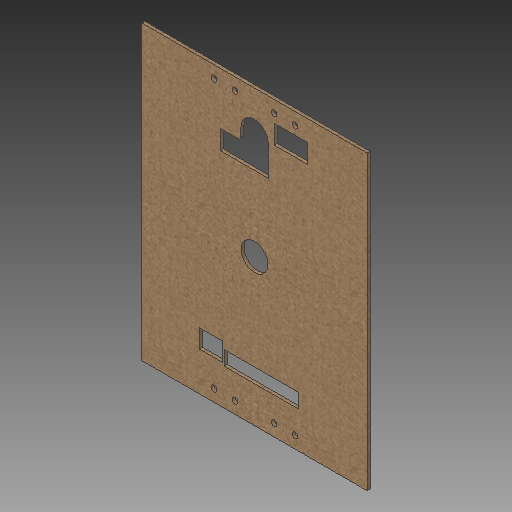
# Autodesk Inventor part: 基板保護2018.8.7
Saved by Autodesk Inventor 2018 (Build 220112000, 112)
## iProperties
Created: 2018-08-07
Part Number: 基板保護2018.8.7
Material: MDF 中密度繊維ボード
Document SubType Name: Modeling
Designer: shun2
Density: 0.8 g/cm^3
Appearance: ダンボール - 段ボール紙
Author: shun2
Autodesk Inventor part; units mm, degrees
(part 1 of 2)
ref_plane "YZ Plane" through (0, 0, 0) normal (1, 0, 0) x (0, 1, 0)
ref_plane "XZ Plane" through (0, 0, 0) normal (0, 1, 0) x (-1, 0, 0)
ref_plane "XY Plane" through (0, 0, 0) normal (0, 0, 1) x (1, 0, 0)
sketch "スケッチ1" plane through (0, 0, 0) normal (0, 0, 1) x (1, 0, 0)
  line L0 (-10, 0) -> (140, 0)
  arc A0 (140, -0.0003) -> (140, 0.0003) centre (140, 0) ccw
  arc A1 (-10, 0.0003) -> (-10, -0.0003) centre (-10, 0) ccw
  line L1 (140, 0) -> (140, 194.7239)
  arc A2 (140.0002, 194.7239) -> (139.9998, 194.7239) centre (140, 194.7239) ccw
  arc A3 (139.9998, 0) -> (140.0002, 0) centre (140, 0) ccw
  line L2 (140, 194.7239) -> (-10, 194.7239)
  arc A4 (-10, 194.7242) -> (-10, 194.7237) centre (-10, 194.72395) ccw
  arc A5 (140, 194.7237) -> (140, 194.7242) centre (140, 194.72395) ccw
  line L3 (-10, 194.7239) -> (-10, 0)
  arc A6 (-10.0002, 0) -> (-9.9998, 0) centre (-10, 0) ccw
  arc A7 (-9.9998, 194.7239) -> (-10.0002, 194.7239) centre (-10, 194.7239) ccw
  arc A8 (65, 88.362) -> (65, 106.362) centre (65, 97.362) ccw
  arc A9 (65, 106.362) -> (65, 88.362) centre (65, 97.362) ccw
  line L4 (89.7664, 26.5952) -> (89.6098, 26.5952)
  arc A10 (89.6098, 26.6143) -> (89.6098, 26.5762) centre (89.6098, 26.59525) ccw
  arc A11 (89.7664, 26.5762) -> (89.7664, 26.6143) centre (89.7664, 26.59525) ccw
  line L5 (89.6098, 26.5952) -> (89.6098, 26.0731)
  arc A12 (89.5907, 26.0731) -> (89.6288, 26.0731) centre (89.60975, 26.0731) ccw
  arc A13 (89.6288, 26.5952) -> (89.5907, 26.5952) centre (89.60975, 26.5952) ccw
  line L6 (89.6098, 26.0731) -> (89.9231, 26.0731)
  arc A14 (89.9231, 26.0541) -> (89.9231, 26.0922) centre (89.9231, 26.07315) ccw
  arc A15 (89.6098, 26.0922) -> (89.6098, 26.0541) centre (89.6098, 26.07315) ccw
  arc A16 (89.9231, 26.0731) -> (90.1319, 26.2819) centre (89.923095, 26.281905) ccw
  arc A17 (89.9231, 26.0922) -> (89.9231, 26.0541) centre (89.9231, 26.07315) ccw
  arc A18 (90.1509, 26.2819) -> (90.1129, 26.2819) centre (90.1319, 26.2819) ccw
  line L7 (90.1319, 26.2819) -> (90.1319, 26.8041)
  arc A19 (90.1509, 26.8041) -> (90.1129, 26.8041) centre (90.1319, 26.8041) ccw
  arc A20 (90.1129, 26.2819) -> (90.1509, 26.2819) centre (90.1319, 26.2819) ccw
  arc A21 (90.1319, 26.8041) -> (89.9231, 27.0129) centre (89.923095, 26.804095) ccw
  arc A22 (90.1129, 26.8041) -> (90.1509, 26.8041) centre (90.1319, 26.8041) ccw
  arc A23 (89.9231, 27.0319) -> (89.9231, 26.9938) centre (89.9231, 27.01285) ccw
  line L8 (89.9231, 27.0129) -> (89.6098, 27.0129)
  arc A24 (89.6098, 27.032) -> (89.6098, 26.9939) centre (89.6098, 27.01295) ccw
  arc A25 (89.9231, 26.9939) -> (89.9231, 27.032) centre (89.9231, 27.01295) ccw
  arc A26 (84.5298, 26.2819) -> (84.7386, 26.0731) centre (84.738605, 26.281905) ccw
  arc A27 (84.5488, 26.2819) -> (84.5107, 26.2819) centre (84.52975, 26.2819) ccw
  arc A28 (84.7386, 26.0541) -> (84.7386, 26.0922) centre (84.7386, 26.07315) ccw
  arc A29 (84.7386, 26.0731) -> (85.0519, 26.2036) centre (84.73865, 26.51431) ccw
  arc A30 (84.7386, 26.0921) -> (84.7386, 26.0541) centre (84.7386, 26.0731) ccw
  arc A31 (85.0654, 26.1902) -> (85.0384, 26.217) centre (85.0519, 26.2036) ccw
  arc A32 (85.0258, 26.8041) -> (84.817, 27.0129) centre (84.816995, 26.804095) ccw
  arc A33 (85.0067, 26.8041) -> (85.0448, 26.8041) centre (85.02575, 26.8041) ccw
  arc A34 (84.817, 27.032) -> (84.817, 26.9939) centre (84.817, 27.01295) ccw
  arc A35 (84.817, 27.0129) -> (84.582, 26.9346) centre (84.816933, 26.621301) ccw
  arc A36 (84.817, 26.9939) -> (84.8169, 27.032) centre (84.81695, 27.01295) ccw
  arc A37 (84.5706, 26.9498) -> (84.5934, 26.9193) centre (84.582, 26.93455) ccw
  arc A38 (84.9214, 26.6213) -> (85.0258, 26.8041) centre (84.813675, 26.804036) ccw
  arc A39 (84.9117, 26.6377) -> (84.931, 26.6049) centre (84.92135, 26.6213) ccw
  arc A40 (85.0448, 26.8041) -> (85.0067, 26.8041) centre (85.02575, 26.8041) ccw
  arc A41 (84.6342, 26.4647) -> (84.5298, 26.2819) centre (84.741925, 26.281964) ccw
  arc A42 (84.6439, 26.4483) -> (84.6245, 26.4811) centre (84.6342, 26.4647) ccw
  arc A43 (84.5107, 26.2819) -> (84.5488, 26.2819) centre (84.52975, 26.2819) ccw
  line L9 (84.6342, 26.4647) -> (84.9214, 26.6213)
  arc A44 (84.9305, 26.6046) -> (84.9123, 26.638) centre (84.9214, 26.6213) ccw
  arc A45 (84.6251, 26.4814) -> (84.6433, 26.448) centre (84.6342, 26.4647) ccw
  line L10 (84.0898, 27.0129) -> (84.0898, 26.0731)
  arc A46 (84.0708, 26.0731) -> (84.1089, 26.0731) centre (84.08985, 26.0731) ccw
  arc A47 (84.1089, 27.0129) -> (84.0708, 27.0129) centre (84.08985, 27.0129) ccw
  line L11 (84.1942, 26.0731) -> (83.9854, 26.0731)
  arc A48 (83.9854, 26.0922) -> (83.9854, 26.0541) centre (83.9854, 26.07315) ccw
  arc A49 (84.1942, 26.0541) -> (84.1942, 26.0922) centre (84.1942, 26.07315) ccw
  line L12 (84.1942, 27.0129) -> (83.9854, 27.0129)
  arc A50 (83.9854, 27.032) -> (83.9854, 26.9939) centre (83.9854, 27.01295) ccw
  arc A51 (84.1942, 26.9939) -> (84.1942, 27.032) centre (84.1942, 27.01295) ccw
  line L13 (83.2234, 26.5952) -> (83.0668, 26.5952)
  arc A52 (83.0668, 26.6143) -> (83.0668, 26.5762) centre (83.0668, 26.59525) ccw
  arc A53 (83.2234, 26.5762) -> (83.2234, 26.6143) centre (83.2234, 26.59525) ccw
  line L14 (83.0668, 26.5952) -> (83.0668, 26.0731)
  arc A54 (83.0477, 26.0731) -> (83.0858, 26.0731) centre (83.06675, 26.0731) ccw
  arc A55 (83.0858, 26.5952) -> (83.0477, 26.5952) centre (83.06675, 26.5952) ccw
  line L15 (83.0668, 26.0731) -> (83.38, 26.0731)
  arc A56 (83.38, 26.0541) -> (83.38, 26.0922) centre (83.38, 26.07315) ccw
  arc A57 (83.0668, 26.0922) -> (83.0668, 26.0541) centre (83.0668, 26.07315) ccw
  arc A58 (83.38, 26.0731) -> (83.5889, 26.2819) centre (83.380045, 26.281955) ccw
  arc A59 (83.38, 26.0922) -> (83.38, 26.0541) centre (83.38, 26.07315) ccw
  arc A60 (83.6079, 26.2819) -> (83.5698, 26.2819) centre (83.58885, 26.2819) ccw
  line L16 (83.5889, 26.2819) -> (83.5889, 26.8041)
  arc A61 (83.6079, 26.8041) -> (83.5698, 26.8041) centre (83.58885, 26.8041) ccw
  arc A62 (83.5698, 26.2819) -> (83.6079, 26.2819) centre (83.58885, 26.2819) ccw
  arc A63 (83.5889, 26.8041) -> (83.38, 27.0129) centre (83.380045, 26.804045) ccw
  arc A64 (83.5698, 26.8041) -> (83.6079, 26.8041) centre (83.58885, 26.8041) ccw
  arc A65 (83.38, 27.0319) -> (83.38, 26.9938) centre (83.38, 27.01285) ccw
  line L17 (83.38, 27.0129) -> (83.0668, 27.0129)
  arc A66 (83.0668, 27.032) -> (83.0668, 26.9939) centre (83.0668, 27.01295) ccw
  arc A67 (83.38, 26.9939) -> (83.38, 27.032) centre (83.38, 27.01295) ccw
  line L18 (83.4433, 173.4847) -> (95.4433, 173.4847)
  arc A68 (95.4433, 173.453) -> (95.4433, 173.5164) centre (95.4433, 173.4847) ccw
  arc A69 (83.4433, 173.5164) -> (83.4433, 173.453) centre (83.4433, 173.4847) ccw
  line L19 (95.4433, 173.4847) -> (95.4433, 176.9847)
  arc A70 (95.4751, 176.9847) -> (95.4116, 176.9847) centre (95.44335, 176.9847) ccw
  arc A71 (95.4116, 173.4847) -> (95.4751, 173.4847) centre (95.44335, 173.4847) ccw
  line L20 (95.4433, 176.9847) -> (83.4433, 176.9847)
  arc A72 (83.4433, 177.0164) -> (83.4433, 176.953) centre (83.4433, 176.9847) ccw
  arc A73 (95.4433, 176.953) -> (95.4433, 177.0164) centre (95.4433, 176.9847) ccw
  line L21 (83.4433, 176.9847) -> (83.4433, 173.4847)
  arc A74 (83.4116, 173.4847) -> (83.4751, 173.4847) centre (83.44335, 173.4847) ccw
  arc A75 (83.4751, 176.9847) -> (83.4116, 176.9847) centre (83.44335, 176.9847) ccw
  line L22 (31.115, 35.941) -> (31.115, 34.544)
  arc A76 (31.0769, 34.544) -> (31.1531, 34.544) centre (31.115, 34.544) ccw
  arc A77 (31.1531, 35.941) -> (31.0769, 35.941) centre (31.115, 35.941) ccw
  line L23 (41.275, 28.448) -> (31.115, 28.448)
  arc A78 (31.115, 28.4861) -> (31.115, 28.4099) centre (31.115, 28.448) ccw
  arc A79 (41.275, 28.4099) -> (41.275, 28.4861) centre (41.275, 28.448) ccw
  line L24 (41.275, 28.448) -> (41.275, 30.226)
  arc A80 (41.3131, 30.226) -> (41.2369, 30.226) centre (41.275, 30.226) ccw
  arc A81 (41.2369, 28.448) -> (41.3131, 28.448) centre (41.275, 28.448) ccw
  line L25 (31.115, 35.941) -> (41.275, 35.941)
  arc A82 (41.275, 35.9029) -> (41.275, 35.9791) centre (41.275, 35.941) ccw
  arc A83 (31.115, 35.9791) -> (31.115, 35.9029) centre (31.115, 35.941) ccw
  line L26 (31.115, 29.337) -> (30.607, 29.21)
  arc A84 (30.5978, 29.247) -> (30.6162, 29.173) centre (30.607, 29.21) ccw
  arc A85 (31.1242, 29.3) -> (31.1058, 29.374) centre (31.115, 29.337) ccw
  line L27 (31.115, 29.337) -> (31.115, 28.448)
  arc A86 (31.0769, 28.448) -> (31.1531, 28.448) centre (31.115, 28.448) ccw
  arc A87 (31.1531, 29.337) -> (31.0769, 29.337) centre (31.115, 29.337) ccw
  line L28 (30.607, 29.21) -> (30.607, 30.353)
  arc A88 (30.6451, 30.353) -> (30.5689, 30.353) centre (30.607, 30.353) ccw
  arc A89 (30.5689, 29.21) -> (30.6451, 29.21) centre (30.607, 29.21) ccw
  line L29 (30.607, 30.353) -> (31.115, 30.226)
  arc A90 (31.1058, 30.189) -> (31.1242, 30.263) centre (31.115, 30.226) ccw
  arc A91 (30.6162, 30.39) -> (30.5978, 30.316) centre (30.607, 30.353) ccw
  line L30 (31.115, 30.226) -> (31.115, 29.337)
  arc A92 (31.0769, 29.337) -> (31.1531, 29.337) centre (31.115, 29.337) ccw
  arc A93 (31.1531, 30.226) -> (31.0769, 30.226) centre (31.115, 30.226) ccw
  line L31 (31.115, 30.226) -> (41.275, 30.226)
  arc A94 (41.275, 30.1879) -> (41.275, 30.2641) centre (41.275, 30.226) ccw
  arc A95 (31.115, 30.2641) -> (31.115, 30.1879) centre (31.115, 30.226) ccw
  line L32 (41.275, 30.226) -> (41.275, 34.544)
  arc A96 (41.3131, 34.544) -> (41.2369, 34.544) centre (41.275, 34.544) ccw
  arc A97 (41.2369, 30.226) -> (41.3131, 30.226) centre (41.275, 30.226) ccw
  line L33 (31.115, 34.544) -> (41.275, 34.544)
  arc A98 (41.275, 34.5059) -> (41.275, 34.5821) centre (41.275, 34.544) ccw
  arc A99 (31.115, 34.5821) -> (31.115, 34.5059) centre (31.115, 34.544) ccw
  line L34 (31.115, 34.544) -> (31.115, 30.226)
  arc A100 (31.0769, 30.226) -> (31.1531, 30.226) centre (31.115, 30.226) ccw
  arc A101 (31.1531, 34.544) -> (31.0769, 34.544) centre (31.115, 34.544) ccw
  line L35 (41.275, 34.544) -> (41.275, 35.941)
  arc A102 (41.3131, 35.941) -> (41.2369, 35.941) centre (41.275, 35.941) ccw
  arc A103 (41.2369, 34.544) -> (41.3131, 34.544) centre (41.275, 34.544) ccw
  line L36 (32.2933, 29.5896) -> (32.0534, 29.7815)
  arc A104 (32.0732, 29.8063) -> (32.0336, 29.7567) centre (32.0534, 29.7815) ccw
  arc A105 (32.2734, 29.5648) -> (32.3131, 29.6144) centre (32.29325, 29.5896) ccw
  line L37 (32.0534, 29.7815) -> (32.0534, 28.9179)
  arc A106 (32.0216, 28.9179) -> (32.0851, 28.9179) centre (32.05335, 28.9179) ccw
  arc A107 (32.0851, 29.7815) -> (32.0216, 29.7815) centre (32.05335, 29.7815) ccw
  line L38 (32.2933, 28.9179) -> (31.8135, 28.9179)
  arc A108 (31.8135, 28.9497) -> (31.8135, 28.8862) centre (31.8135, 28.91795) ccw
  arc A109 (32.2933, 28.8862) -> (32.2933, 28.9497) centre (32.2933, 28.91795) ccw
  arc A110 (37.1094, 29.7815) -> (36.8935, 29.5656) centre (37.109405, 29.565595) ccw
  arc A111 (37.1094, 29.7498) -> (37.1094, 29.8133) centre (37.1094, 29.78155) ccw
  arc A112 (36.8618, 29.5656) -> (36.9253, 29.5656) centre (36.89355, 29.5656) ccw
  arc A113 (37.3733, 29.5896) -> (37.1094, 29.7815) centre (37.109427, 29.50413) ccw
  arc A114 (37.3431, 29.5798) -> (37.4035, 29.5994) centre (37.3733, 29.5896) ccw
  arc A115 (37.1094, 29.8132) -> (37.1094, 29.7498) centre (37.1094, 29.7815) ccw
  arc A116 (36.8935, 29.5656) -> (36.9655, 29.3977) centre (37.125339, 29.565631) ccw
  arc A117 (36.9252, 29.5656) -> (36.8618, 29.5656) centre (36.8935, 29.5656) ccw
  arc A118 (36.9436, 29.3747) -> (36.9874, 29.4207) centre (36.9655, 29.3977) ccw
  line L39 (36.9655, 29.3977) -> (37.3733, 28.9179)
  arc A119 (37.3491, 28.8973) -> (37.3975, 28.9385) centre (37.3733, 28.9179) ccw
  arc A120 (36.9897, 29.4182) -> (36.9413, 29.3771) centre (36.9655, 29.39765) ccw
  line L40 (37.3733, 28.9179) -> (36.8935, 28.9179)
  arc A121 (36.8935, 28.9497) -> (36.8935, 28.8862) centre (36.8935, 28.91795) ccw
  arc A122 (37.3733, 28.8862) -> (37.3733, 28.9497) centre (37.3733, 28.91795) ccw
  arc A123 (38.7096, 28.829) -> (38.7096, 29.845) centre (38.7096, 29.337) ccw
  arc A124 (38.7096, 29.845) -> (38.7096, 28.829) centre (38.7096, 29.337) ccw
  arc A125 (33.6804, 28.829) -> (33.6804, 29.845) centre (33.6804, 29.337) ccw
  arc A126 (33.6804, 29.845) -> (33.6804, 28.829) centre (33.6804, 29.337) ccw
  line L41 (47.085, 27.46) -> (48.355, 27.46)
  arc A127 (48.355, 27.4219) -> (48.355, 27.4981) centre (48.355, 27.46) ccw
  arc A128 (47.085, 27.4981) -> (47.085, 27.4219) centre (47.085, 27.46) ccw
  line L42 (48.355, 27.46) -> (48.99, 28.095)
  arc A129 (49.0169, 28.0681) -> (48.9631, 28.1219) centre (48.99, 28.095) ccw
  arc A130 (48.3281, 27.4869) -> (48.3819, 27.4331) centre (48.355, 27.46) ccw
  line L43 (48.99, 29.365) -> (48.355, 30)
  arc A131 (48.3819, 30.0269) -> (48.3281, 29.9731) centre (48.355, 30) ccw
  arc A132 (48.9631, 29.3381) -> (49.0169, 29.3919) centre (48.99, 29.365) ccw
  line L44 (48.99, 28.095) -> (49.625, 27.46)
  arc A133 (49.5981, 27.4331) -> (49.6519, 27.4869) centre (49.625, 27.46) ccw
  arc A134 (49.0169, 28.1219) -> (48.9631, 28.0681) centre (48.99, 28.095) ccw
  line L45 (49.625, 27.46) -> (50.895, 27.46)
  arc A135 (50.895, 27.4219) -> (50.895, 27.4981) centre (50.895, 27.46) ccw
  arc A136 (49.625, 27.4981) -> (49.625, 27.4219) centre (49.625, 27.46) ccw
  line L46 (50.895, 27.46) -> (51.53, 28.095)
  arc A137 (51.5569, 28.0681) -> (51.5031, 28.1219) centre (51.53, 28.095) ccw
  arc A138 (50.8681, 27.4869) -> (50.9219, 27.4331) centre (50.895, 27.46) ccw
  line L47 (51.53, 29.365) -> (50.895, 30)
  arc A139 (50.9219, 30.0269) -> (50.8681, 29.9731) centre (50.895, 30) ccw
  arc A140 (51.5031, 29.3381) -> (51.5569, 29.3919) centre (51.53, 29.365) ccw
  line L48 (50.895, 30) -> (49.625, 30)
  arc A141 (49.625, 30.0381) -> (49.625, 29.9619) centre (49.625, 30) ccw
  arc A142 (50.895, 29.9619) -> (50.895, 30.0381) centre (50.895, 30) ccw
  line L49 (49.625, 30) -> (48.99, 29.365)
  arc A143 (48.9631, 29.3919) -> (49.0169, 29.3381) centre (48.99, 29.365) ccw
  arc A144 (49.6519, 29.9731) -> (49.5981, 30.0269) centre (49.625, 30) ccw
  line L50 (46.45, 28.095) -> (46.45, 29.365)
  arc A145 (46.4881, 29.365) -> (46.4119, 29.365) centre (46.45, 29.365) ccw
  arc A146 (46.4119, 28.095) -> (46.4881, 28.095) centre (46.45, 28.095) ccw
  line L51 (47.085, 27.46) -> (46.45, 28.095)
  arc A147 (46.4769, 28.1219) -> (46.4231, 28.0681) centre (46.45, 28.095) ccw
  arc A148 (47.0581, 27.4331) -> (47.1119, 27.4869) centre (47.085, 27.46) ccw
  line L52 (46.45, 29.365) -> (47.085, 30)
  arc A149 (47.1119, 29.9731) -> (47.0581, 30.0269) centre (47.085, 30) ccw
  arc A150 (46.4231, 29.3919) -> (46.4769, 29.3381) centre (46.45, 29.365) ccw
  line L53 (48.355, 30) -> (47.085, 30)
  arc A151 (47.085, 30.0381) -> (47.085, 29.9619) centre (47.085, 30) ccw
  arc A152 (48.355, 29.9619) -> (48.355, 30.0381) centre (48.355, 30) ccw
  line L54 (51.53, 28.095) -> (52.165, 27.46)
  arc A153 (52.1381, 27.4331) -> (52.1919, 27.4869) centre (52.165, 27.46) ccw
  arc A154 (51.5569, 28.1219) -> (51.5031, 28.0681) centre (51.53, 28.095) ccw
  line L55 (52.165, 27.46) -> (53.435, 27.46)
  arc A155 (53.435, 27.4219) -> (53.435, 27.4981) centre (53.435, 27.46) ccw
  arc A156 (52.165, 27.4981) -> (52.165, 27.4219) centre (52.165, 27.46) ccw
  line L56 (53.435, 27.46) -> (54.07, 28.095)
  arc A157 (54.0969, 28.0681) -> (54.0431, 28.1219) centre (54.07, 28.095) ccw
  arc A158 (53.4081, 27.4869) -> (53.4619, 27.4331) centre (53.435, 27.46) ccw
  line L57 (54.07, 29.365) -> (53.435, 30)
  arc A159 (53.4619, 30.0269) -> (53.4081, 29.9731) centre (53.435, 30) ccw
  arc A160 (54.0431, 29.3381) -> (54.0969, 29.3919) centre (54.07, 29.365) ccw
  line L58 (53.435, 30) -> (52.165, 30)
  arc A161 (52.165, 30.0381) -> (52.165, 29.9619) centre (52.165, 30) ccw
  arc A162 (53.435, 29.9619) -> (53.435, 30.0381) centre (53.435, 30) ccw
  line L59 (52.165, 30) -> (51.53, 29.365)
  arc A163 (51.5031, 29.3919) -> (51.5569, 29.3381) centre (51.53, 29.365) ccw
  arc A164 (52.1919, 29.9731) -> (52.1381, 30.0269) centre (52.165, 30) ccw
  line L60 (54.705, 27.46) -> (55.975, 27.46)
  arc A165 (55.975, 27.4219) -> (55.975, 27.4981) centre (55.975, 27.46) ccw
  arc A166 (54.705, 27.4981) -> (54.705, 27.4219) centre (54.705, 27.46) ccw
  line L61 (55.975, 27.46) -> (56.61, 28.095)
  arc A167 (56.6369, 28.0681) -> (56.5831, 28.1219) centre (56.61, 28.095) ccw
  arc A168 (55.9481, 27.4869) -> (56.0019, 27.4331) centre (55.975, 27.46) ccw
  line L62 (56.61, 29.365) -> (55.975, 30)
  arc A169 (56.0019, 30.0269) -> (55.9481, 29.9731) centre (55.975, 30) ccw
  arc A170 (56.5831, 29.3381) -> (56.6369, 29.3919) centre (56.61, 29.365) ccw
  line L63 (56.61, 28.095) -> (57.245, 27.46)
  arc A171 (57.2181, 27.4331) -> (57.2719, 27.4869) centre (57.245, 27.46) ccw
  arc A172 (56.6369, 28.1219) -> (56.5831, 28.0681) centre (56.61, 28.095) ccw
  line L64 (57.245, 27.46) -> (58.515, 27.46)
  arc A173 (58.515, 27.4219) -> (58.515, 27.4981) centre (58.515, 27.46) ccw
  arc A174 (57.245, 27.4981) -> (57.245, 27.4219) centre (57.245, 27.46) ccw
  line L65 (58.515, 27.46) -> (59.15, 28.095)
  arc A175 (59.1769, 28.0681) -> (59.1231, 28.1219) centre (59.15, 28.095) ccw
  arc A176 (58.4881, 27.4869) -> (58.5419, 27.4331) centre (58.515, 27.46) ccw
  line L66 (59.15, 29.365) -> (58.515, 30)
  arc A177 (58.5419, 30.0269) -> (58.4881, 29.9731) centre (58.515, 30) ccw
  arc A178 (59.1231, 29.3381) -> (59.1769, 29.3919) centre (59.15, 29.365) ccw
  line L67 (58.515, 30) -> (57.245, 30)
  arc A179 (57.245, 30.0381) -> (57.245, 29.9619) centre (57.245, 30) ccw
  arc A180 (58.515, 29.9619) -> (58.515, 30.0381) centre (58.515, 30) ccw
  line L68 (57.245, 30) -> (56.61, 29.365)
  arc A181 (56.5831, 29.3919) -> (56.6369, 29.3381) centre (56.61, 29.365) ccw
  arc A182 (57.2719, 29.9731) -> (57.2181, 30.0269) centre (57.245, 30) ccw
  line L69 (54.705, 27.46) -> (54.07, 28.095)
  arc A183 (54.0969, 28.1219) -> (54.0431, 28.0681) centre (54.07, 28.095) ccw
  arc A184 (54.6781, 27.4331) -> (54.7319, 27.4869) centre (54.705, 27.46) ccw
  line L70 (54.07, 29.365) -> (54.705, 30)
  arc A185 (54.7319, 29.9731) -> (54.6781, 30.0269) centre (54.705, 30) ccw
  arc A186 (54.0431, 29.3919) -> (54.0969, 29.3381) centre (54.07, 29.365) ccw
  line L71 (55.975, 30) -> (54.705, 30)
  arc A187 (54.705, 30.0381) -> (54.705, 29.9619) centre (54.705, 30) ccw
  arc A188 (55.975, 29.9619) -> (55.975, 30.0381) centre (55.975, 30) ccw
  line L72 (59.15, 28.095) -> (59.785, 27.46)
  arc A189 (59.7581, 27.4331) -> (59.8119, 27.4869) centre (59.785, 27.46) ccw
  arc A190 (59.1769, 28.1219) -> (59.1231, 28.0681) centre (59.15, 28.095) ccw
  line L73 (59.785, 27.46) -> (61.055, 27.46)
  arc A191 (61.055, 27.4219) -> (61.055, 27.4981) centre (61.055, 27.46) ccw
  arc A192 (59.785, 27.4981) -> (59.785, 27.4219) centre (59.785, 27.46) ccw
  line L74 (61.055, 27.46) -> (61.69, 28.095)
  arc A193 (61.7169, 28.0681) -> (61.6631, 28.1219) centre (61.69, 28.095) ccw
  arc A194 (61.0281, 27.4869) -> (61.0819, 27.4331) centre (61.055, 27.46) ccw
  line L75 (61.69, 29.365) -> (61.055, 30)
  arc A195 (61.0819, 30.0269) -> (61.0281, 29.9731) centre (61.055, 30) ccw
  arc A196 (61.6631, 29.3381) -> (61.7169, 29.3919) centre (61.69, 29.365) ccw
  line L76 (61.055, 30) -> (59.785, 30)
  arc A197 (59.785, 30.0381) -> (59.785, 29.9619) centre (59.785, 30) ccw
  arc A198 (61.055, 29.9619) -> (61.055, 30.0381) centre (61.055, 30) ccw
  line L77 (59.785, 30) -> (59.15, 29.365)
  arc A199 (59.1231, 29.3919) -> (59.1769, 29.3381) centre (59.15, 29.365) ccw
  arc A200 (59.8119, 29.9731) -> (59.7581, 30.0269) centre (59.785, 30) ccw
  line L78 (62.325, 27.46) -> (63.595, 27.46)
  arc A201 (63.595, 27.4219) -> (63.595, 27.4981) centre (63.595, 27.46) ccw
  arc A202 (62.325, 27.4981) -> (62.325, 27.4219) centre (62.325, 27.46) ccw
  line L79 (63.595, 27.46) -> (64.23, 28.095)
  arc A203 (64.2569, 28.0681) -> (64.2031, 28.1219) centre (64.23, 28.095) ccw
  arc A204 (63.5681, 27.4869) -> (63.6219, 27.4331) centre (63.595, 27.46) ccw
  line L80 (64.23, 29.365) -> (63.595, 30)
  arc A205 (63.6219, 30.0269) -> (63.5681, 29.9731) centre (63.595, 30) ccw
  arc A206 (64.2031, 29.3381) -> (64.2569, 29.3919) centre (64.23, 29.365) ccw
  line L81 (64.23, 28.095) -> (64.865, 27.46)
  arc A207 (64.8381, 27.4331) -> (64.8919, 27.4869) centre (64.865, 27.46) ccw
  arc A208 (64.2569, 28.1219) -> (64.2031, 28.0681) centre (64.23, 28.095) ccw
  line L82 (64.865, 27.46) -> (66.135, 27.46)
  arc A209 (66.135, 27.4219) -> (66.135, 27.4981) centre (66.135, 27.46) ccw
  arc A210 (64.865, 27.4981) -> (64.865, 27.4219) centre (64.865, 27.46) ccw
  line L83 (66.135, 27.46) -> (66.77, 28.095)
  arc A211 (66.7969, 28.0681) -> (66.7431, 28.1219) centre (66.77, 28.095) ccw
  arc A212 (66.1081, 27.4869) -> (66.1619, 27.4331) centre (66.135, 27.46) ccw
  line L84 (66.77, 29.365) -> (66.135, 30)
  arc A213 (66.1619, 30.0269) -> (66.1081, 29.9731) centre (66.135, 30) ccw
  arc A214 (66.7431, 29.3381) -> (66.7969, 29.3919) centre (66.77, 29.365) ccw
  line L85 (66.135, 30) -> (64.865, 30)
  arc A215 (64.865, 30.0381) -> (64.865, 29.9619) centre (64.865, 30) ccw
  arc A216 (66.135, 29.9619) -> (66.135, 30.0381) centre (66.135, 30) ccw
  line L86 (64.865, 30) -> (64.23, 29.365)
  arc A217 (64.2031, 29.3919) -> (64.2569, 29.3381) centre (64.23, 29.365) ccw
  arc A218 (64.8919, 29.9731) -> (64.8381, 30.0269) centre (64.865, 30) ccw
  line L87 (62.325, 27.46) -> (61.69, 28.095)
  arc A219 (61.7169, 28.1219) -> (61.6631, 28.0681) centre (61.69, 28.095) ccw
  arc A220 (62.2981, 27.4331) -> (62.3519, 27.4869) centre (62.325, 27.46) ccw
  line L88 (61.69, 29.365) -> (62.325, 30)
  arc A221 (62.3519, 29.9731) -> (62.2981, 30.0269) centre (62.325, 30) ccw
  arc A222 (61.6631, 29.3919) -> (61.7169, 29.3381) centre (61.69, 29.365) ccw
  line L89 (63.595, 30) -> (62.325, 30)
  arc A223 (62.325, 30.0381) -> (62.325, 29.9619) centre (62.325, 30) ccw
  arc A224 (63.595, 29.9619) -> (63.595, 30.0381) centre (63.595, 30) ccw
  line L90 (66.77, 28.095) -> (67.405, 27.46)
  arc A225 (67.3781, 27.4331) -> (67.4319, 27.4869) centre (67.405, 27.46) ccw
  arc A226 (66.7969, 28.1219) -> (66.7431, 28.0681) centre (66.77, 28.095) ccw
  line L91 (67.405, 27.46) -> (68.675, 27.46)
  arc A227 (68.675, 27.4219) -> (68.675, 27.4981) centre (68.675, 27.46) ccw
  arc A228 (67.405, 27.4981) -> (67.405, 27.4219) centre (67.405, 27.46) ccw
  line L92 (68.675, 27.46) -> (69.31, 28.095)
  arc A229 (69.3369, 28.0681) -> (69.2831, 28.1219) centre (69.31, 28.095) ccw
  arc A230 (68.6481, 27.4869) -> (68.7019, 27.4331) centre (68.675, 27.46) ccw
  line L93 (69.31, 29.365) -> (68.675, 30)
  arc A231 (68.7019, 30.0269) -> (68.6481, 29.9731) centre (68.675, 30) ccw
  arc A232 (69.2831, 29.3381) -> (69.3369, 29.3919) centre (69.31, 29.365) ccw
  line L94 (68.675, 30) -> (67.405, 30)
  arc A233 (67.405, 30.0381) -> (67.405, 29.9619) centre (67.405, 30) ccw
  arc A234 (68.675, 29.9619) -> (68.675, 30.0381) centre (68.675, 30) ccw
  line L95 (67.405, 30) -> (66.77, 29.365)
  arc A235 (66.7431, 29.3919) -> (66.7969, 29.3381) centre (66.77, 29.365) ccw
  arc A236 (67.4319, 29.9731) -> (67.3781, 30.0269) centre (67.405, 30) ccw
  line L96 (69.945, 27.46) -> (71.215, 27.46)
  arc A237 (71.215, 27.4219) -> (71.215, 27.4981) centre (71.215, 27.46) ccw
  arc A238 (69.945, 27.4981) -> (69.945, 27.4219) centre (69.945, 27.46) ccw
  line L97 (71.215, 27.46) -> (71.85, 28.095)
  arc A239 (71.8769, 28.0681) -> (71.8231, 28.1219) centre (71.85, 28.095) ccw
  arc A240 (71.1881, 27.4869) -> (71.2419, 27.4331) centre (71.215, 27.46) ccw
  line L98 (71.85, 29.365) -> (71.215, 30)
  arc A241 (71.2419, 30.0269) -> (71.1881, 29.9731) centre (71.215, 30) ccw
  arc A242 (71.8231, 29.3381) -> (71.8769, 29.3919) centre (71.85, 29.365) ccw
  line L99 (71.85, 28.095) -> (72.485, 27.46)
  arc A243 (72.4581, 27.4331) -> (72.5119, 27.4869) centre (72.485, 27.46) ccw
  arc A244 (71.8769, 28.1219) -> (71.8231, 28.0681) centre (71.85, 28.095) ccw
  line L100 (72.485, 27.46) -> (73.755, 27.46)
  arc A245 (73.755, 27.4219) -> (73.755, 27.4981) centre (73.755, 27.46) ccw
  arc A246 (72.485, 27.4981) -> (72.485, 27.4219) centre (72.485, 27.46) ccw
  line L101 (73.755, 27.46) -> (74.39, 28.095)
  arc A247 (74.4169, 28.0681) -> (74.3631, 28.1219) centre (74.39, 28.095) ccw
  arc A248 (73.7281, 27.4869) -> (73.7819, 27.4331) centre (73.755, 27.46) ccw
  line L102 (74.39, 29.365) -> (73.755, 30)
  arc A249 (73.7819, 30.0269) -> (73.7281, 29.9731) centre (73.755, 30) ccw
  arc A250 (74.3631, 29.3381) -> (74.4169, 29.3919) centre (74.39, 29.365) ccw
  line L103 (73.755, 30) -> (72.485, 30)
  arc A251 (72.485, 30.0381) -> (72.485, 29.9619) centre (72.485, 30) ccw
  arc A252 (73.755, 29.9619) -> (73.755, 30.0381) centre (73.755, 30) ccw
  line L104 (72.485, 30) -> (71.85, 29.365)
  arc A253 (71.8231, 29.3919) -> (71.8769, 29.3381) centre (71.85, 29.365) ccw
  arc A254 (72.5119, 29.9731) -> (72.4581, 30.0269) centre (72.485, 30) ccw
  line L105 (69.945, 27.46) -> (69.31, 28.095)
  arc A255 (69.3369, 28.1219) -> (69.2831, 28.0681) centre (69.31, 28.095) ccw
  arc A256 (69.9181, 27.4331) -> (69.9719, 27.4869) centre (69.945, 27.46) ccw
  line L106 (69.31, 29.365) -> (69.945, 30)
  arc A257 (69.9719, 29.9731) -> (69.9181, 30.0269) centre (69.945, 30) ccw
  arc A258 (69.2831, 29.3919) -> (69.3369, 29.3381) centre (69.31, 29.365) ccw
  line L107 (71.215, 30) -> (69.945, 30)
  arc A259 (69.945, 30.0381) -> (69.945, 29.9619) centre (69.945, 30) ccw
  arc A260 (71.215, 29.9619) -> (71.215, 30.0381) centre (71.215, 30) ccw
  line L108 (74.39, 28.095) -> (75.025, 27.46)
  arc A261 (74.9981, 27.4331) -> (75.0519, 27.4869) centre (75.025, 27.46) ccw
  arc A262 (74.4169, 28.1219) -> (74.3631, 28.0681) centre (74.39, 28.095) ccw
  line L109 (75.025, 27.46) -> (76.295, 27.46)
  arc A263 (76.295, 27.4219) -> (76.295, 27.4981) centre (76.295, 27.46) ccw
  arc A264 (75.025, 27.4981) -> (75.025, 27.4219) centre (75.025, 27.46) ccw
  line L110 (76.295, 27.46) -> (76.93, 28.095)
  arc A265 (76.9569, 28.0681) -> (76.9031, 28.1219) centre (76.93, 28.095) ccw
  arc A266 (76.2681, 27.4869) -> (76.3219, 27.4331) centre (76.295, 27.46) ccw
  line L111 (76.93, 29.365) -> (76.295, 30)
  arc A267 (76.3219, 30.0269) -> (76.2681, 29.9731) centre (76.295, 30) ccw
  arc A268 (76.9031, 29.3381) -> (76.9569, 29.3919) centre (76.93, 29.365) ccw
  line L112 (76.295, 30) -> (75.025, 30)
  arc A269 (75.025, 30.0381) -> (75.025, 29.9619) centre (75.025, 30) ccw
  arc A270 (76.295, 29.9619) -> (76.295, 30.0381) centre (76.295, 30) ccw
  line L113 (75.025, 30) -> (74.39, 29.365)
  arc A271 (74.3631, 29.3919) -> (74.4169, 29.3381) centre (74.39, 29.365) ccw
  arc A272 (75.0519, 29.9731) -> (74.9981, 30.0269) centre (75.025, 30) ccw
  line L114 (76.93, 28.095) -> (77.565, 27.46)
  arc A273 (77.5381, 27.4331) -> (77.5919, 27.4869) centre (77.565, 27.46) ccw
  arc A274 (76.9569, 28.1219) -> (76.9031, 28.0681) centre (76.93, 28.095) ccw
  line L115 (77.565, 27.46) -> (78.835, 27.46)
  arc A275 (78.835, 27.4219) -> (78.835, 27.4981) centre (78.835, 27.46) ccw
  arc A276 (77.565, 27.4981) -> (77.565, 27.4219) centre (77.565, 27.46) ccw
  line L116 (79.47, 28.095) -> (79.47, 29.365)
  arc A277 (79.5081, 29.365) -> (79.4319, 29.365) centre (79.47, 29.365) ccw
  arc A278 (79.4319, 28.095) -> (79.5081, 28.095) centre (79.47, 28.095) ccw
  line L117 (78.835, 27.46) -> (79.47, 28.095)
  arc A279 (79.4969, 28.0681) -> (79.4431, 28.1219) centre (79.47, 28.095) ccw
  arc A280 (78.8081, 27.4869) -> (78.8619, 27.4331) centre (78.835, 27.46) ccw
  line L118 (79.47, 29.365) -> (78.835, 30)
  arc A281 (78.8619, 30.0269) -> (78.8081, 29.9731) centre (78.835, 30) ccw
  arc A282 (79.4431, 29.3381) -> (79.4969, 29.3919) centre (79.47, 29.365) ccw
  line L119 (78.835, 30) -> (77.565, 30)
  arc A283 (77.565, 30.0381) -> (77.565, 29.9619) centre (77.565, 30) ccw
  arc A284 (78.835, 29.9619) -> (78.835, 30.0381) centre (78.835, 30) ccw
  line L120 (77.565, 30) -> (76.93, 29.365)
  arc A285 (76.9031, 29.3919) -> (76.9569, 29.3381) centre (76.93, 29.365) ccw
  arc A286 (77.5919, 29.9731) -> (77.5381, 30.0269) centre (77.565, 30) ccw
  line L121 (47.9105, 31.3335) -> (47.593, 31.5875)
  arc A287 (47.6128, 31.6123) -> (47.5732, 31.5627) centre (47.593, 31.5875) ccw
  arc A288 (47.8907, 31.3087) -> (47.9303, 31.3583) centre (47.9105, 31.3335) ccw
  line L122 (47.593, 31.5875) -> (47.593, 30.4445)
  arc A289 (47.5613, 30.4445) -> (47.6248, 30.4445) centre (47.59305, 30.4445) ccw
  arc A290 (47.6248, 31.5875) -> (47.5613, 31.5875) centre (47.59305, 31.5875) ccw
  line L123 (47.9105, 30.4445) -> (47.2755, 30.4445)
  arc A291 (47.2755, 30.4763) -> (47.2755, 30.4128) centre (47.2755, 30.44455) ccw
  arc A292 (47.9105, 30.4128) -> (47.9105, 30.4763) centre (47.9105, 30.44455) ccw
  line L124 (78.8985, 26.7615) -> (78.581, 27.0155)
  arc A293 (78.6008, 27.0403) -> (78.5612, 26.9907) centre (78.581, 27.0155) ccw
  arc A294 (78.8787, 26.7367) -> (78.9183, 26.7863) centre (78.8985, 26.7615) ccw
  line L125 (78.581, 27.0155) -> (78.581, 25.8725)
  arc A295 (78.5493, 25.8725) -> (78.6128, 25.8725) centre (78.58105, 25.8725) ccw
  arc A296 (78.6128, 27.0155) -> (78.5493, 27.0155) centre (78.58105, 27.0155) ccw
  line L126 (78.8985, 25.8725) -> (78.2635, 25.8725)
  arc A297 (78.2635, 25.9043) -> (78.2635, 25.8408) centre (78.2635, 25.87255) ccw
  arc A298 (78.8985, 25.8408) -> (78.8985, 25.9043) centre (78.8985, 25.87255) ccw
  line L127 (77.7555, 25.8725) -> (77.438, 25.8725)
  arc A299 (77.438, 25.9043) -> (77.438, 25.8408) centre (77.438, 25.87255) ccw
  arc A300 (77.7555, 25.8408) -> (77.7555, 25.9043) centre (77.7555, 25.87255) ccw
  arc A301 (77.438, 26.5075) -> (77.438, 25.8725) centre (77.438, 26.19) ccw
  arc A302 (77.438, 26.4758) -> (77.438, 26.5392) centre (77.438, 26.5075) ccw
  arc A303 (77.438, 25.8408) -> (77.438, 25.9043) centre (77.438, 25.87255) ccw
  line L128 (77.7555, 27.0155) -> (77.3745, 27.0155)
  arc A304 (77.3745, 27.0473) -> (77.3745, 26.9838) centre (77.3745, 27.01555) ccw
  arc A305 (77.7555, 26.9838) -> (77.7555, 27.0473) centre (77.7555, 27.01555) ccw
  arc A306 (77.3745, 27.0155) -> (77.3745, 26.5075) centre (77.3745, 26.7615) ccw
  arc A307 (77.3745, 26.9838) -> (77.3745, 27.0473) centre (77.3745, 27.01555) ccw
  arc A308 (77.3745, 26.4758) -> (77.3745, 26.5392) centre (77.3745, 26.5075) ccw
  line L129 (77.3745, 26.5075) -> (77.6285, 26.5075)
  arc A309 (77.6285, 26.4758) -> (77.6285, 26.5392) centre (77.6285, 26.5075) ccw
  arc A310 (77.3745, 26.5392) -> (77.3745, 26.4758) centre (77.3745, 26.5075) ccw
  line L130 (92.13, 32.69) -> (92.13, 27.61)
  arc A311 (92.0983, 27.61) -> (92.1618, 27.61) centre (92.13005, 27.61) ccw
  arc A312 (92.1618, 32.69) -> (92.0983, 32.69) centre (92.13005, 32.69) ccw
  line L131 (92.13, 27.61) -> (90.86, 27.61)
  arc A313 (90.86, 27.6418) -> (90.86, 27.5783) centre (90.86, 27.61005) ccw
  arc A314 (92.13, 27.5783) -> (92.13, 27.6418) centre (92.13, 27.61005) ccw
  line L132 (90.86, 27.61) -> (83.24, 27.61)
  arc A315 (83.24, 27.6418) -> (83.24, 27.5783) centre (83.24, 27.61005) ccw
  arc A316 (90.86, 27.5783) -> (90.86, 27.6418) centre (90.86, 27.61005) ccw
  line L133 (83.24, 27.61) -> (81.97, 27.61)
  arc A317 (81.97, 27.6418) -> (81.97, 27.5783) centre (81.97, 27.61005) ccw
  arc A318 (83.24, 27.5783) -> (83.24, 27.6418) centre (83.24, 27.61005) ccw
  line L134 (81.97, 27.61) -> (81.97, 32.69)
  arc A319 (82.0018, 32.69) -> (81.9382, 32.69) centre (81.97, 32.69) ccw
  arc A320 (81.9382, 27.61) -> (82.0018, 27.61) centre (81.97, 27.61) ccw
  line L135 (81.97, 32.69) -> (92.13, 32.69)
  arc A321 (92.13, 32.6583) -> (92.13, 32.7218) centre (92.13, 32.69005) ccw
  arc A322 (81.97, 32.7218) -> (81.97, 32.6583) centre (81.97, 32.69005) ccw
  line L136 (90.86, 27.61) -> (90.86, 28.88)
  arc A323 (90.8918, 28.88) -> (90.8282, 28.88) centre (90.86, 28.88) ccw
  arc A324 (90.8282, 27.61) -> (90.8918, 27.61) centre (90.86, 27.61) ccw
  line L137 (90.86, 28.88) -> (83.24, 28.88)
  arc A325 (83.24, 28.9118) -> (83.24, 28.8483) centre (83.24, 28.88005) ccw
  arc A326 (90.86, 28.8483) -> (90.86, 28.9118) centre (90.86, 28.88005) ccw
  line L138 (83.24, 28.88) -> (83.24, 27.61)
  arc A327 (83.2083, 27.61) -> (83.2718, 27.61) centre (83.24005, 27.61) ccw
  arc A328 (83.2718, 28.88) -> (83.2083, 28.88) centre (83.24005, 28.88) ccw
  arc A329 (93.9433, 174.5922) -> (93.9433, 175.1172) centre (93.9433, 174.8547) ccw
  arc A330 (93.9433, 175.1172) -> (93.9433, 174.5922) centre (93.9433, 174.8547) ccw
  arc A331 (93.9433, 174.5922) -> (93.9433, 175.1172) centre (93.9433, 174.8547) ccw
  arc A332 (93.9433, 175.1172) -> (93.9433, 174.5922) centre (93.9433, 174.8547) ccw
  arc A333 (92.4433, 174.5922) -> (92.4433, 175.1172) centre (92.4433, 174.8547) ccw
  arc A334 (92.4433, 175.1172) -> (92.4433, 174.5922) centre (92.4433, 174.8547) ccw
  arc A335 (92.4433, 174.5922) -> (92.4433, 175.1172) centre (92.4433, 174.8547) ccw
  arc A336 (92.4433, 175.1172) -> (92.4433, 174.5922) centre (92.4433, 174.8547) ccw
  arc A337 (90.9433, 174.5922) -> (90.9433, 175.1172) centre (90.9433, 174.8547) ccw
  arc A338 (90.9433, 175.1172) -> (90.9433, 174.5922) centre (90.9433, 174.8547) ccw
  arc A339 (90.9433, 174.5922) -> (90.9433, 175.1172) centre (90.9433, 174.8547) ccw
  arc A340 (90.9433, 175.1172) -> (90.9433, 174.5922) centre (90.9433, 174.8547) ccw
  arc A341 (89.4433, 174.5922) -> (89.4433, 175.1172) centre (89.4433, 174.8547) ccw
  arc A342 (89.4433, 175.1172) -> (89.4433, 174.5922) centre (89.4433, 174.8547) ccw
  arc A343 (89.4433, 174.5922) -> (89.4433, 175.1172) centre (89.4433, 174.8547) ccw
  arc A344 (89.4433, 175.1172) -> (89.4433, 174.5922) centre (89.4433, 174.8547) ccw
  arc A345 (87.9433, 174.5922) -> (87.9433, 175.1172) centre (87.9433, 174.8547) ccw
  arc A346 (87.9433, 175.1172) -> (87.9433, 174.5922) centre (87.9433, 174.8547) ccw
  arc A347 (87.9433, 174.5922) -> (87.9433, 175.1172) centre (87.9433, 174.8547) ccw
  arc A348 (87.9433, 175.1172) -> (87.9433, 174.5922) centre (87.9433, 174.8547) ccw
  arc A349 (86.4433, 174.5922) -> (86.4433, 175.1172) centre (86.4433, 174.8547) ccw
  arc A350 (86.4433, 175.1172) -> (86.4433, 174.5922) centre (86.4433, 174.8547) ccw
  arc A351 (86.4433, 174.5922) -> (86.4433, 175.1172) centre (86.4433, 174.8547) ccw
  arc A352 (86.4433, 175.1172) -> (86.4433, 174.5922) centre (86.4433, 174.8547) ccw
  arc A353 (84.9433, 174.5922) -> (84.9433, 175.1172) centre (84.9433, 174.8547) ccw
  arc A354 (84.9433, 175.1172) -> (84.9433, 174.5922) centre (84.9433, 174.8547) ccw
  arc A355 (84.9433, 174.5922) -> (84.9433, 175.1172) centre (84.9433, 174.8547) ccw
  arc A356 (84.9433, 175.1172) -> (84.9433, 174.5922) centre (84.9433, 174.8547) ccw
  line L139 (35.695, 31.885) -> (36.695, 31.885)
  line L140 (36.695, 31.885) -> (36.695, 32.885)
  line L141 (36.695, 32.885) -> (35.695, 32.885)
  line L142 (35.695, 32.885) -> (35.695, 31.885)
  line L143 (33.6804, 33.3756) -> (33.6804, 31.3944)
  arc A357 (33.1851, 31.3944) -> (34.1757, 31.3944) centre (33.6804, 31.3944) ccw
  arc A358 (34.1757, 33.3756) -> (33.1851, 33.3756) centre (33.6804, 33.3756) ccw
  line L144 (33.6804, 33.3756) -> (33.6804, 31.3944)
  arc A359 (33.1851, 31.3944) -> (34.1757, 31.3944) centre (33.6804, 31.3944) ccw
  arc A360 (34.1757, 33.3756) -> (33.1851, 33.3756) centre (33.6804, 33.3756) ccw
  line L145 (38.7096, 33.3756) -> (38.7096, 31.3944)
  arc A361 (38.2143, 31.3944) -> (39.2049, 31.3944) centre (38.7096, 31.3944) ccw
  arc A362 (39.2049, 33.3756) -> (38.2143, 33.3756) centre (38.7096, 33.3756) ccw
  line L146 (38.7096, 33.3756) -> (38.7096, 31.3944)
  arc A363 (38.2143, 31.3944) -> (39.2049, 31.3944) centre (38.7096, 31.3944) ccw
  arc A364 (39.2049, 33.3756) -> (38.2143, 33.3756) centre (38.7096, 33.3756) ccw
  line L147 (50.006, 28.476) -> (50.514, 28.476)
  line L148 (50.514, 28.476) -> (50.514, 28.984)
  line L149 (50.514, 28.984) -> (50.006, 28.984)
  line L150 (50.006, 28.984) -> (50.006, 28.476)
  line L151 (47.466, 28.476) -> (47.974, 28.476)
  line L152 (47.974, 28.476) -> (47.974, 28.984)
  line L153 (47.974, 28.984) -> (47.466, 28.984)
  line L154 (47.466, 28.984) -> (47.466, 28.476)
  line L155 (52.546, 28.476) -> (53.054, 28.476)
  line L156 (53.054, 28.476) -> (53.054, 28.984)
  line L157 (53.054, 28.984) -> (52.546, 28.984)
  line L158 (52.546, 28.984) -> (52.546, 28.476)
  line L159 (57.626, 28.476) -> (58.134, 28.476)
  line L160 (58.134, 28.476) -> (58.134, 28.984)
  line L161 (58.134, 28.984) -> (57.626, 28.984)
  line L162 (57.626, 28.984) -> (57.626, 28.476)
  line L163 (55.086, 28.476) -> (55.594, 28.476)
  line L164 (55.594, 28.476) -> (55.594, 28.984)
  line L165 (55.594, 28.984) -> (55.086, 28.984)
  line L166 (55.086, 28.984) -> (55.086, 28.476)
  line L167 (60.166, 28.476) -> (60.674, 28.476)
  line L168 (60.674, 28.476) -> (60.674, 28.984)
  line L169 (60.674, 28.984) -> (60.166, 28.984)
  line L170 (60.166, 28.984) -> (60.166, 28.476)
  line L171 (65.246, 28.476) -> (65.754, 28.476)
  line L172 (65.754, 28.476) -> (65.754, 28.984)
  line L173 (65.754, 28.984) -> (65.246, 28.984)
  line L174 (65.246, 28.984) -> (65.246, 28.476)
  line L175 (62.706, 28.476) -> (63.214, 28.476)
  line L176 (63.214, 28.476) -> (63.214, 28.984)
  line L177 (63.214, 28.984) -> (62.706, 28.984)
  line L178 (62.706, 28.984) -> (62.706, 28.476)
  line L179 (67.786, 28.476) -> (68.294, 28.476)
  line L180 (68.294, 28.476) -> (68.294, 28.984)
  line L181 (68.294, 28.984) -> (67.786, 28.984)
  line L182 (67.786, 28.984) -> (67.786, 28.476)
  line L183 (72.866, 28.476) -> (73.374, 28.476)
  line L184 (73.374, 28.476) -> (73.374, 28.984)
  line L185 (73.374, 28.984) -> (72.866, 28.984)
  line L186 (72.866, 28.984) -> (72.866, 28.476)
  line L187 (70.326, 28.476) -> (70.834, 28.476)
  line L188 (70.834, 28.476) -> (70.834, 28.984)
  line L189 (70.834, 28.984) -> (70.326, 28.984)
  line L190 (70.326, 28.984) -> (70.326, 28.476)
  line L191 (75.406, 28.476) -> (75.914, 28.476)
  line L192 (75.914, 28.476) -> (75.914, 28.984)
  line L193 (75.914, 28.984) -> (75.406, 28.984)
  line L194 (75.406, 28.984) -> (75.406, 28.476)
  line L195 (77.946, 28.476) -> (78.454, 28.476)
  line L196 (78.454, 28.476) -> (78.454, 28.984)
  line L197 (78.454, 28.984) -> (77.946, 28.984)
  line L198 (77.946, 28.984) -> (77.946, 28.476)
  arc A365 (47.339, 28.73) -> (48.101, 28.73) centre (47.72, 28.73) ccw
  arc A366 (48.101, 28.73) -> (47.339, 28.73) centre (47.72, 28.73) ccw
  arc A367 (47.339, 28.73) -> (48.101, 28.73) centre (47.72, 28.73) ccw
  arc A368 (48.101, 28.73) -> (47.339, 28.73) centre (47.72, 28.73) ccw
  arc A369 (49.879, 28.73) -> (50.641, 28.73) centre (50.26, 28.73) ccw
  arc A370 (50.641, 28.73) -> (49.879, 28.73) centre (50.26, 28.73) ccw
  arc A371 (49.879, 28.73) -> (50.641, 28.73) centre (50.26, 28.73) ccw
  arc A372 (50.641, 28.73) -> (49.879, 28.73) centre (50.26, 28.73) ccw
  arc A373 (52.419, 28.73) -> (53.181, 28.73) centre (52.8, 28.73) ccw
  arc A374 (53.181, 28.73) -> (52.419, 28.73) centre (52.8, 28.73) ccw
  arc A375 (52.419, 28.73) -> (53.181, 28.73) centre (52.8, 28.73) ccw
  arc A376 (53.181, 28.73) -> (52.419, 28.73) centre (52.8, 28.73) ccw
  arc A377 (54.959, 28.73) -> (55.721, 28.73) centre (55.34, 28.73) ccw
  arc A378 (55.721, 28.73) -> (54.959, 28.73) centre (55.34, 28.73) ccw
  arc A379 (54.959, 28.73) -> (55.721, 28.73) centre (55.34, 28.73) ccw
  arc A380 (55.721, 28.73) -> (54.959, 28.73) centre (55.34, 28.73) ccw
  arc A381 (57.499, 28.73) -> (58.261, 28.73) centre (57.88, 28.73) ccw
  arc A382 (58.261, 28.73) -> (57.499, 28.73) centre (57.88, 28.73) ccw
  arc A383 (57.499, 28.73) -> (58.261, 28.73) centre (57.88, 28.73) ccw
  arc A384 (58.261, 28.73) -> (57.499, 28.73) centre (57.88, 28.73) ccw
  arc A385 (60.039, 28.73) -> (60.801, 28.73) centre (60.42, 28.73) ccw
  arc A386 (60.801, 28.73) -> (60.039, 28.73) centre (60.42, 28.73) ccw
  arc A387 (60.039, 28.73) -> (60.801, 28.73) centre (60.42, 28.73) ccw
  arc A388 (60.801, 28.73) -> (60.039, 28.73) centre (60.42, 28.73) ccw
  arc A389 (62.579, 28.73) -> (63.341, 28.73) centre (62.96, 28.73) ccw
  arc A390 (63.341, 28.73) -> (62.579, 28.73) centre (62.96, 28.73) ccw
  arc A391 (62.579, 28.73) -> (63.341, 28.73) centre (62.96, 28.73) ccw
  arc A392 (63.341, 28.73) -> (62.579, 28.73) centre (62.96, 28.73) ccw
  arc A393 (65.119, 28.73) -> (65.881, 28.73) centre (65.5, 28.73) ccw
  arc A394 (65.881, 28.73) -> (65.119, 28.73) centre (65.5, 28.73) ccw
  arc A395 (65.119, 28.73) -> (65.881, 28.73) centre (65.5, 28.73) ccw
  arc A396 (65.881, 28.73) -> (65.119, 28.73) centre (65.5, 28.73) ccw
  arc A397 (67.659, 28.73) -> (68.421, 28.73) centre (68.04, 28.73) ccw
  arc A398 (68.421, 28.73) -> (67.659, 28.73) centre (68.04, 28.73) ccw
  arc A399 (67.659, 28.73) -> (68.421, 28.73) centre (68.04, 28.73) ccw
  arc A400 (68.421, 28.73) -> (67.659, 28.73) centre (68.04, 28.73) ccw
  arc A401 (70.199, 28.73) -> (70.961, 28.73) centre (70.58, 28.73) ccw
  arc A402 (70.961, 28.73) -> (70.199, 28.73) centre (70.58, 28.73) ccw
  arc A403 (70.199, 28.73) -> (70.961, 28.73) centre (70.58, 28.73) ccw
  arc A404 (70.961, 28.73) -> (70.199, 28.73) centre (70.58, 28.73) ccw
  arc A405 (72.739, 28.73) -> (73.501, 28.73) centre (73.12, 28.73) ccw
  arc A406 (73.501, 28.73) -> (72.739, 28.73) centre (73.12, 28.73) ccw
  arc A407 (72.739, 28.73) -> (73.501, 28.73) centre (73.12, 28.73) ccw
  arc A408 (73.501, 28.73) -> (72.739, 28.73) centre (73.12, 28.73) ccw
  arc A409 (75.279, 28.73) -> (76.041, 28.73) centre (75.66, 28.73) ccw
  arc A410 (76.041, 28.73) -> (75.279, 28.73) centre (75.66, 28.73) ccw
  arc A411 (75.279, 28.73) -> (76.041, 28.73) centre (75.66, 28.73) ccw
  arc A412 (76.041, 28.73) -> (75.279, 28.73) centre (75.66, 28.73) ccw
  arc A413 (77.819, 28.73) -> (78.581, 28.73) centre (78.2, 28.73) ccw
  arc A414 (78.581, 28.73) -> (77.819, 28.73) centre (78.2, 28.73) ccw
  arc A415 (77.819, 28.73) -> (78.581, 28.73) centre (78.2, 28.73) ccw
  arc A416 (78.581, 28.73) -> (77.819, 28.73) centre (78.2, 28.73) ccw
  arc A417 (89.59, 30.6) -> (89.59, 29.7) centre (89.59, 30.15) ccw
  arc A418 (89.59, 29.7) -> (89.59, 30.6) centre (89.59, 30.15) ccw
  arc A419 (89.59, 30.6) -> (89.59, 29.7) centre (89.59, 30.15) ccw
  arc A420 (89.59, 29.7) -> (89.59, 30.6) centre (89.59, 30.15) ccw
  arc A421 (87.05, 30.6) -> (87.05, 29.7) centre (87.05, 30.15) ccw
  arc A422 (87.05, 29.7) -> (87.05, 30.6) centre (87.05, 30.15) ccw
  arc A423 (87.05, 30.6) -> (87.05, 29.7) centre (87.05, 30.15) ccw
  arc A424 (87.05, 29.7) -> (87.05, 30.6) centre (87.05, 30.15) ccw
  arc A425 (84.51, 30.6) -> (84.51, 29.7) centre (84.51, 30.15) ccw
  arc A426 (84.51, 29.7) -> (84.51, 30.6) centre (84.51, 30.15) ccw
  arc A427 (84.51, 30.6) -> (84.51, 29.7) centre (84.51, 30.15) ccw
  arc A428 (84.51, 29.7) -> (84.51, 30.6) centre (84.51, 30.15) ccw
  arc A429 (52, 184.7239) -> (52, 188.7239) centre (52, 186.7239) ccw
  arc A430 (52, 188.7239) -> (52, 184.7239) centre (52, 186.7239) ccw
  arc A431 (52, 184.7239) -> (52, 188.7239) centre (52, 186.7239) ccw
  arc A432 (52, 188.7239) -> (52, 184.7239) centre (52, 186.7239) ccw
  arc A433 (52, 6) -> (52, 10) centre (52, 8) ccw
  arc A434 (52, 10) -> (52, 6) centre (52, 8) ccw
  arc A435 (52, 6) -> (52, 10) centre (52, 8) ccw
  arc A436 (52, 10) -> (52, 6) centre (52, 8) ccw
  arc A437 (78, 6) -> (78, 10) centre (78, 8) ccw
  arc A438 (78, 10) -> (78, 6) centre (78, 8) ccw
  arc A439 (78, 6) -> (78, 10) centre (78, 8) ccw
  arc A440 (78, 10) -> (78, 6) centre (78, 8) ccw
  arc A441 (38, 6) -> (38, 10) centre (38, 8) ccw
  arc A442 (38, 10) -> (38, 6) centre (38, 8) ccw
  arc A443 (38, 6) -> (38, 10) centre (38, 8) ccw
  arc A444 (38, 10) -> (38, 6) centre (38, 8) ccw
  arc A445 (92, 6) -> (92, 10) centre (92, 8) ccw
  arc A446 (92, 10) -> (92, 6) centre (92, 8) ccw
  arc A447 (92, 6) -> (92, 10) centre (92, 8) ccw
  arc A448 (92, 10) -> (92, 6) centre (92, 8) ccw
  arc A449 (92, 184.7239) -> (92, 188.7239) centre (92, 186.7239) ccw
  arc A450 (92, 188.7239) -> (92, 184.7239) centre (92, 186.7239) ccw
  arc A451 (92, 184.7239) -> (92, 188.7239) centre (92, 186.7239) ccw
  arc A452 (92, 188.7239) -> (92, 184.7239) centre (92, 186.7239) ccw
  arc A453 (78, 184.7239) -> (78, 188.7239) centre (78, 186.7239) ccw
  arc A454 (78, 188.7239) -> (78, 184.7239) centre (78, 186.7239) ccw
  arc A455 (78, 184.7239) -> (78, 188.7239) centre (78, 186.7239) ccw
  arc A456 (78, 188.7239) -> (78, 184.7239) centre (78, 186.7239) ccw
  arc A457 (38, 184.7239) -> (38, 188.7239) centre (38, 186.7239) ccw
  arc A458 (38, 188.7239) -> (38, 184.7239) centre (38, 186.7239) ccw
  arc A459 (38, 184.7239) -> (38, 188.7239) centre (38, 186.7239) ccw
  arc A460 (38, 188.7239) -> (38, 184.7239) centre (38, 186.7239) ccw
  line L199 (-10.0002, 194.7239) -> (140.0002, 194.7239)
  line L200 (140.0002, 194.7239) -> (140.0002, 0)
  line L201 (140.0002, 0) -> (-10.0002, 0)
  line L202 (-10.0002, 0) -> (-10.0002, 194.7239)
  line L203 (78, 180.99093) -> (100.51742, 180.99093)
  line L204 (100.51742, 180.99093) -> (100.51742, 168.379005)
  line L205 (100.51742, 168.379005) -> (78, 168.379005)
  line L206 (78, 168.379005) -> (78, 180.99093)
  line L207 (44.73875, 33.8709) -> (94, 33.8709)
  line L208 (94, 33.8709) -> (94, 24.202729)
  line L209 (94, 24.202729) -> (44.73875, 24.202729)
  line L210 (44.73875, 24.202729) -> (44.73875, 33.8709)
  line L211 (28.37271, 38.147158) -> (43.54174, 38.147158)
  line L212 (43.54174, 38.147158) -> (43.54174, 25.87255)
  line L213 (43.54174, 25.87255) -> (28.37271, 25.87255)
  line L214 (28.37271, 25.87255) -> (28.37271, 38.147158)
  circle A461 centre (65, 97.362) radius 9
  circle A462 centre (38, 186.7239) radius 2
  circle A463 centre (52, 186.7239) radius 2
  circle A464 centre (78, 186.7239) radius 2
  circle A465 centre (92, 186.7239) radius 2
  circle A466 centre (38, 8) radius 2
  circle A467 centre (52, 8) radius 2
  circle A468 centre (78, 8) radius 2
  circle A469 centre (92, 8) radius 2
  line L215 (74.3631, 160.034298) -> (74.3631, 147.261346)
  arc A470 (73.999457, 167.822801) -> (65, 176.7239) centre (65, 167.7239) ccw
  arc A471 (56.515, 158.2293) -> (56.515, 158.3055) centre (56.515, 158.2674) ccw
  arc A472 (56.5531, 158.2674) -> (56.4769, 158.2674) centre (56.515, 158.2674) ccw
  arc A473 (57.0138, 156.3254) -> (57.0322, 156.3994) centre (57.023, 156.3624) ccw
  line L216 (56.515, 157.3784) -> (56.515, 158.2674)
  arc A474 (56.9849, 156.3624) -> (57.0611, 156.3624) centre (57.023, 156.3624) ccw
  arc A475 (56.4769, 156.4894) -> (56.5531, 156.4894) centre (56.515, 156.4894) ccw
  arc A476 (65, 176.7239) -> (56, 167.7239) centre (65, 167.7239) ccw
  arc A477 (56.5242, 156.5264) -> (56.5058, 156.4524) centre (56.515, 156.4894) ccw
  arc A478 (57.0611, 157.5054) -> (56.9849, 157.5054) centre (57.023, 157.5054) ccw
  arc A479 (56.5058, 157.4154) -> (56.5242, 157.3414) centre (56.515, 157.3784) ccw
  arc A480 (46.3169, 156.4894) -> (46.3931, 156.4894) centre (46.355, 156.4894) ccw
  line L217 (46.355, 158.2674) -> (46.355, 156.4894)
  arc A481 (46.3931, 158.2674) -> (46.3169, 158.2674) centre (46.355, 158.2674) ccw
  arc A482 (46.355, 158.3055) -> (46.355, 158.2293) centre (46.355, 158.2674) ccw
  line L218 (56.515, 150.7744) -> (56.515, 152.1714)
  arc A483 (56.5531, 152.1714) -> (56.4769, 152.1714) centre (56.515, 152.1714) ccw
  line L219 (46.355, 158.2674) -> (56.515, 158.2674)
  line L220 (56.515, 150.7744) -> (46.355, 150.7744)
  arc A484 (46.355, 150.8125) -> (46.355, 150.7363) centre (46.355, 150.7744) ccw
  arc A485 (56.4769, 150.7744) -> (56.5531, 150.7744) centre (56.515, 150.7744) ccw
  arc A486 (56.515, 150.7363) -> (56.515, 150.8125) centre (56.515, 150.7744) ccw
  arc A487 (46.3169, 152.1714) -> (46.3931, 152.1714) centre (46.355, 152.1714) ccw
  arc A488 (65.645, 153.9) -> (65.645, 154.8) centre (65.645, 154.35) ccw
  arc A489 (65.645, 153.9) -> (65.645, 154.8) centre (65.645, 154.35) ccw
  arc A490 (63.105, 153.9) -> (63.105, 154.8) centre (63.105, 154.35) ccw
  arc A491 (63.105, 153.9) -> (63.105, 154.8) centre (63.105, 154.35) ccw
  arc A492 (63.105, 154.8) -> (63.105, 153.9) centre (63.105, 154.35) ccw
  arc A493 (63.105, 154.8) -> (63.105, 153.9) centre (63.105, 154.35) ccw
  arc A494 (46.3931, 156.4894) -> (46.3169, 156.4894) centre (46.355, 156.4894) ccw
  arc A495 (56.5531, 156.4894) -> (56.4769, 156.4894) centre (56.515, 156.4894) ccw
  line L221 (56.515, 156.4894) -> (56.515, 157.3784)
  arc A496 (56.4769, 157.3784) -> (56.5531, 157.3784) centre (56.515, 157.3784) ccw
  arc A497 (56.5531, 157.3784) -> (56.4769, 157.3784) centre (56.515, 157.3784) ccw
  line L222 (57.023, 157.5054) -> (57.023, 156.3624)
  arc A498 (57.0322, 157.4684) -> (57.0138, 157.5424) centre (57.023, 157.5054) ccw
  line L223 (56.515, 157.3784) -> (57.023, 157.5054)
  arc A499 (46.3931, 152.1714) -> (46.3169, 152.1714) centre (46.355, 152.1714) ccw
  arc A500 (46.355, 152.2095) -> (46.355, 152.1333) centre (46.355, 152.1714) ccw
  line L224 (46.355, 152.1714) -> (46.355, 150.7744)
  line L225 (56.515, 152.1714) -> (46.355, 152.1714)
  arc A501 (56.4769, 152.1714) -> (56.5531, 152.1714) centre (56.515, 152.1714) ccw
  line L226 (46.355, 156.4894) -> (46.355, 152.1714)
  line L227 (56.515, 156.4894) -> (46.355, 156.4894)
  line L228 (56.515, 152.1714) -> (56.515, 156.4894)